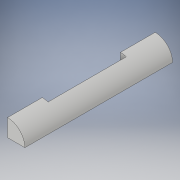
# Autodesk Inventor part: topOfStairs_025_notch
Saved by Autodesk Inventor 2019.1 (Build 231200000, 200)
## iProperties
Created: 2018-09-03
Part Number: topOfStairs_025_notch
Material: Generic
Document SubType Name: Modeling
Designer: steele
Density: 1 g/cm^3
Appearance: Default
Author: steele
Autodesk Inventor part; units mm, degrees
ref_plane "YZ Plane" through (0, 0, 0) normal (1, 0, 0) x (0, 1, 0)
ref_plane "XZ Plane" through (0, 0, 0) normal (0, 1, 0) x (-1, 0, 0)
ref_plane "XY Plane" through (0, 0, 0) normal (0, 0, 1) x (1, 0, 0)
sketch "Sketch1" plane through (0, 0, 0) normal (0, 0, 1) x (1, 0, 0)
  arc A0 (19.05, 0) -> (0, 19.05) centre (0, 0) ccw
  line L0 (0, 19.05) -> (0, 0)
  line L1 (0, 0) -> (19.05, 0)
  dimension "d0" = 38.1
  constraints: 4 end point, 2 point on circle, 1 centre point, 1 coincident, 1 perpendicular, 1 vertical
  measures "d0" diameter of A0
extrude "Extrusion1" add sketch "Sketch1" along normal mid plane 161.925
sketch "Sketch2" plane through (0, 0, 80.9625) normal (0, -1, 0) x (1, 0, 0)
  line L0 (0, -38.1) -> (6.35, -38.1)
  line L1 (6.35, -38.1) -> (6.35, -123.825)
  line L2 (6.35, -123.825) -> (0, -123.825)
  line L3 (0, -123.825) -> (0, -38.1)
  line L4 (19.05, -161.925) -> (0, -161.925) projected
  line L5 (0, -161.925) -> (0, 0) projected
  point P0 (0, -80.9625)
  dimension "d3" = 85.725
  dimension "d4" = 38.1
  dimension "d5" = 6.35
  constraints: 8 end point, 2 parallel, 1 collinear, 1 horizontal, 1 perpendicular
  measures "d3" distance of L0.end L1.end
  measures "d4" distance between parallel lines of L2 L4
  measures "d5" distance of L0.start L0.end
extrude "Extrusion2" cut sketch "Sketch2" against normal through all
equation "\"d0\" = cornerRoundType"
equation "\"d1\" = lengthOfPart"
equation "\"d3\" = notchCutout"
equation "\"d4\" = bottomLength"
equation "\"d5\" = notchDepth"
equation "\"cornerRoundType\" = 38.1"
equation "\"notchCutout\" = 85.725"
equation "\"bottomLength\" = 38.1"
equation "\"lengthOfPart\" = 2 * bottomLength + notchCutout"
equation "\"notchDepth\" = 6.35"
body "Solid1"
